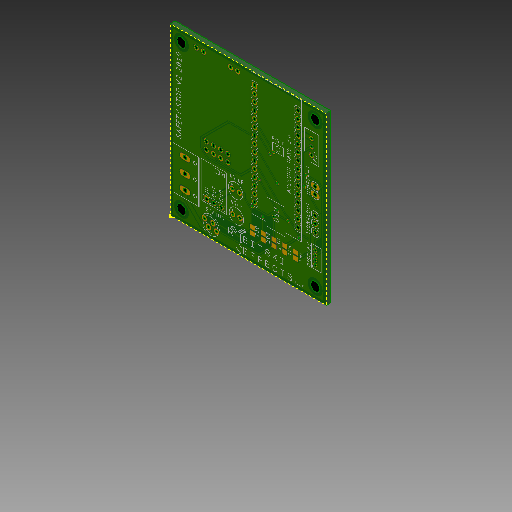
# Autodesk Inventor part: estop v2.brd_Outline
Saved by Autodesk Inventor 2019 (Build 230136000, 136)
## iProperties
Created: 2019-10-02
Part Number: estop v2.brd_Outline
Material: Generic
Document SubType Name: Modeling
Designer: rybit
Density: 1 g/cm^3
Appearance: Board Outline
Author: rybit
Autodesk Inventor part; units mm, degrees
ref_plane "YZ Plane" through (0, 0, 0) normal (1, 0, 0) x (0, 1, 0)
ref_plane "XZ Plane" through (0, 0, 0) normal (0, 1, 0) x (-1, 0, 0)
ref_plane "XY Plane" through (0, 0, 0) normal (0, 0, 1) x (1, 0, 0)
sketch "Sketch1" plane through (0, 0, 0) normal (0, 0, 1) x (1, 0, 0)
  line L0 (0, 0) -> (54.61, 0)
  line L1 (54.61, 0) -> (54.61, 58.42)
  line L2 (54.61, 58.42) -> (0, 58.42)
  line L3 (0, 58.42) -> (0, 0)
  circle A0 centre (49.53, 43.18) radius 0.375
  circle A1 centre (49.53, 45.72) radius 0.375
  circle A2 centre (49.53, 48.26) radius 0.375
  circle A3 centre (21.59, 19.05) radius 0.405
  circle A4 centre (24.13, 19.05) radius 0.405
  circle A5 centre (21.84, 11.43) radius 0.405
  circle A6 centre (24.38, 11.43) radius 0.405
  circle A7 centre (50.8, 10.45) radius 0.35
  circle A8 centre (50.8, 11.95) radius 0.35
  circle A9 centre (50.8, 13.45) radius 0.35
  circle A10 centre (50.8, 14.95) radius 0.35
  circle A11 centre (50.8, 31.75) radius 0.51
  circle A12 centre (50.8, 34.29) radius 0.51
  circle A13 centre (29.46, 54.36) radius 0.5
  circle A14 centre (29.46, 51.82) radius 0.5
  circle A15 centre (29.46, 49.28) radius 0.5
  circle A16 centre (29.46, 46.74) radius 0.5
  circle A17 centre (29.46, 44.2) radius 0.5
  circle A18 centre (29.46, 41.66) radius 0.5
  circle A19 centre (29.46, 39.12) radius 0.5
  circle A20 centre (29.46, 36.58) radius 0.5
  circle A21 centre (29.46, 34.04) radius 0.5
  circle A22 centre (29.46, 31.5) radius 0.5
  circle A23 centre (29.46, 28.96) radius 0.5
  circle A24 centre (29.46, 26.42) radius 0.5
  circle A25 centre (29.46, 23.88) radius 0.5
  circle A26 centre (29.46, 21.34) radius 0.5
  circle A27 centre (29.46, 18.8) radius 0.5
  circle A28 centre (44.7, 54.36) radius 0.5
  circle A29 centre (44.7, 51.82) radius 0.5
  circle A30 centre (44.7, 49.28) radius 0.5
  circle A31 centre (44.7, 46.74) radius 0.5
  circle A32 centre (44.7, 44.2) radius 0.5
  circle A33 centre (44.7, 41.66) radius 0.5
  circle A34 centre (44.7, 39.12) radius 0.5
  circle A35 centre (44.7, 36.58) radius 0.5
  circle A36 centre (44.7, 34.04) radius 0.5
  circle A37 centre (44.7, 31.5) radius 0.5
  circle A38 centre (44.7, 28.96) radius 0.5
  circle A39 centre (44.7, 26.42) radius 0.5
  circle A40 centre (44.7, 23.88) radius 0.5
  circle A41 centre (44.7, 21.34) radius 0.5
  circle A42 centre (44.7, 18.8) radius 0.5
  circle A43 centre (50.8, 25.4) radius 0.51
  circle A44 centre (50.8, 22.86) radius 0.51
  circle A45 centre (50.8, 20.32) radius 0.51
  circle A46 centre (11.81, 5.16) radius 0.4
  circle A47 centre (13.34, 3.22) radius 0.4
  circle A48 centre (14.86, 5.16) radius 0.4
  circle A49 centre (16.13, 3.22) radius 0.4
  circle A50 centre (15.04, 26.34) radius 0.5
  circle A51 centre (15.04, 28.88) radius 0.5
  circle A52 centre (12.5, 26.34) radius 0.5
  circle A53 centre (20.12, 28.88) radius 0.5
  circle A54 centre (20.12, 26.34) radius 0.5
  circle A55 centre (17.58, 28.88) radius 0.5
  circle A56 centre (23.54, 55.69) radius 0.5
  circle A57 centre (21, 55.69) radius 0.5
  circle A58 centre (11.54, 55.69) radius 0.5
  circle A59 centre (9, 55.69) radius 0.5
  circle A60 centre (17.58, 26.34) radius 0.5
  circle A61 centre (12.5, 28.88) radius 0.5
  circle A62 centre (12.7, 11.43) radius 0.5
  circle A63 centre (15.24, 11.43) radius 0.5
  circle A64 centre (17.78, 11.43) radius 0.5
  circle A65 centre (5.06, 20.24) radius 0.595
  circle A66 centre (5.06, 15.24) radius 0.595
  circle A67 centre (5.06, 10.24) radius 0.595
  circle A68 centre (3.81, 54.61) radius 1.5875
  circle A69 centre (3.81, 3.81) radius 1.5875
  circle A70 centre (50.8, 54.61) radius 1.5875
  circle A71 centre (50.8, 3.81) radius 1.5875
  circle A72 centre (32.385, 15.875) radius 0.254
  circle A73 centre (34.925, 36.195) radius 0.254
  circle A74 centre (36.195, 17.78) radius 0.254
  circle A75 centre (36.195, 37.465) radius 0.254
  circle A76 centre (46.99, 32.385) radius 0.254
  circle A77 centre (47.625, 36.195) radius 0.254
  circle A78 centre (45.085, 15.875) radius 0.254
  circle A79 centre (37.465, 28.575) radius 0.254
  circle A80 centre (31.115, 26.67) radius 0.254
  circle A81 centre (37.465, 20.32) radius 0.254
  circle A82 centre (28.575, 17.145) radius 0.254
  circle A83 centre (41.275, 19.05) radius 0.254
  constraints: 84 centre point, 8 end point
extrude "estop v2.brd_Outline" add sketch "Sketch1" along normal blind 1.6383
sketch "Sketch2" plane through (0, 0, 1.6383) normal (0, 0, 1) x (1, 0, 0)
  point P0 (0, 0)
sketch "Sketch3" plane through (0, 0, 1.6383) normal (0, 0, 1) x (1, 0, 0)
  line L0 (0, 0) -> (0, 58.374) construction
  line L1 (0, 58.374) -> (54.5957, 58.374) construction
  line L2 (54.5957, 58.374) -> (54.5957, 0) construction
  line L3 (54.5957, 0) -> (0, 0) construction
  constraints: 2 other
body "Solid1"
